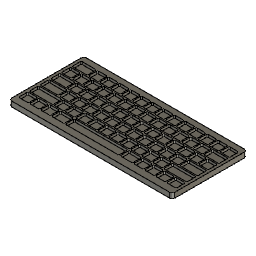
Week 3 HW Keyboard (Autodesk Fusion 360 design; units mm, degrees)
Autodesk Fusion 360 part; units mm, degrees
(part 1 of 2)
sketch "Key outlines" plane through (0, 0, 0) normal (0, 0, 1) x (1, 0, 0)
  spline S0 degree 3 poles (7.7819, -17.5295) (7.6676, -17.5295) (7.5745, -17.4364) (7.5745, -17.3224) knots 0 0 0 0 1 1 1 1
  line L0 (7.5745, -17.3224) -> (7.5745, -15.9198)
  spline S1 degree 3 poles (7.5745, -15.9198) (7.5745, -15.8059) (7.6676, -15.7127) (7.7819, -15.7127) knots 0 0 0 0 1 1 1 1
  line L1 (7.7819, -15.7127) -> (9.2724, -15.7127)
  spline S2 degree 3 poles (9.2724, -15.7127) (9.3864, -15.7127) (9.4795, -15.8059) (9.4795, -15.9198) knots 0 0 0 0 1 1 1 1
  line L2 (9.4795, -15.9198) -> (9.4795, -17.3224)
  spline S3 degree 3 poles (9.4795, -17.3224) (9.4795, -17.4364) (9.3864, -17.5295) (9.2724, -17.5295) knots 0 0 0 0 1 1 1 1
  line L3 (9.2724, -17.5295) -> (7.7819, -17.5295)
  spline S4 degree 3 poles (9.9243, -17.5295) (9.81, -17.5295) (9.7169, -17.4364) (9.7169, -17.3224) knots 0 0 0 0 1 1 1 1
  line L4 (9.7169, -17.3224) -> (9.7169, -15.9198)
  spline S5 degree 3 poles (9.7169, -15.9198) (9.7169, -15.8059) (9.81, -15.7127) (9.9243, -15.7127) knots 0 0 0 0 1 1 1 1
  line L5 (9.9243, -15.7127) -> (11.4148, -15.7127)
  spline S6 degree 3 poles (11.4148, -15.7127) (11.5291, -15.7127) (11.6219, -15.8059) (11.6219, -15.9198) knots 0 0 0 0 1 1 1 1
  line L6 (11.6219, -15.9198) -> (11.6219, -17.3224)
  spline S7 degree 3 poles (11.6219, -17.3224) (11.6219, -17.4364) (11.5291, -17.5295) (11.4148, -17.5295) knots 0 0 0 0 1 1 1 1
  line L7 (11.4148, -17.5295) -> (9.9243, -17.5295)
  spline S8 degree 3 poles (12.0668, -17.5295) (11.9525, -17.5295) (11.8593, -17.4364) (11.8593, -17.3224) knots 0 0 0 0 1 1 1 1
  line L8 (11.8593, -17.3224) -> (11.8593, -15.9198)
  spline S9 degree 3 poles (11.8593, -15.9198) (11.8593, -15.8059) (11.9525, -15.7127) (12.0668, -15.7127) knots 0 0 0 0 1 1 1 1
  line L9 (12.0668, -15.7127) -> (13.5572, -15.7127)
  spline S10 degree 3 poles (13.5572, -15.7127) (13.6716, -15.7127) (13.7643, -15.8059) (13.7643, -15.9198) knots 0 0 0 0 1 1 1 1
  line L10 (13.7643, -15.9198) -> (13.7643, -17.3224)
  spline S11 degree 3 poles (13.7643, -17.3224) (13.7643, -17.4364) (13.6716, -17.5295) (13.5572, -17.5295) knots 0 0 0 0 1 1 1 1
  line L11 (13.5572, -17.5295) -> (12.0668, -17.5295)
  spline S12 degree 3 poles (14.2092, -17.5295) (14.0949, -17.5295) (14.0017, -17.4364) (14.0017, -17.3224) knots 0 0 0 0 1 1 1 1
  line L12 (14.0017, -17.3224) -> (14.0017, -15.9198)
  spline S13 degree 3 poles (14.0017, -15.9198) (14.0017, -15.8059) (14.0949, -15.7127) (14.2092, -15.7127) knots 0 0 0 0 1 1 1 1
  line L13 (14.2092, -15.7127) -> (15.6997, -15.7127)
  spline S14 degree 3 poles (15.6997, -15.7127) (15.814, -15.7127) (15.9067, -15.8059) (15.9067, -15.9198) knots 0 0 0 0 1 1 1 1
  line L14 (15.9067, -15.9198) -> (15.9067, -17.3224)
  spline S15 degree 3 poles (15.9067, -17.3224) (15.9067, -17.4364) (15.814, -17.5295) (15.6997, -17.5295) knots 0 0 0 0 1 1 1 1
  line L15 (15.6997, -17.5295) -> (14.2092, -17.5295)
  spline S16 degree 3 poles (16.3516, -17.5295) (16.2373, -17.5295) (16.1445, -17.4364) (16.1445, -17.3224) knots 0 0 0 0 1 1 1 1
  line L16 (16.1445, -17.3224) -> (16.1445, -15.9198)
  spline S17 degree 3 poles (16.1445, -15.9198) (16.1445, -15.8059) (16.2373, -15.7127) (16.3516, -15.7127) knots 0 0 0 0 1 1 1 1
  line L17 (16.3516, -15.7127) -> (17.8421, -15.7127)
  spline S18 degree 3 poles (17.8421, -15.7127) (17.9564, -15.7127) (18.0492, -15.8059) (18.0492, -15.9198) knots 0 0 0 0 1 1 1 1
  line L18 (18.0492, -15.9198) -> (18.0492, -17.3224)
  spline S19 degree 3 poles (18.0492, -17.3224) (18.0492, -17.4364) (17.9564, -17.5295) (17.8421, -17.5295) knots 0 0 0 0 1 1 1 1
  line L19 (17.8421, -17.5295) -> (16.3516, -17.5295)
  spline S20 degree 3 poles (18.494, -17.5295) (18.3797, -17.5295) (18.2869, -17.4364) (18.2869, -17.3224) knots 0 0 0 0 1 1 1 1
  line L20 (18.2869, -17.3224) -> (18.2869, -15.9198)
  spline S21 degree 3 poles (18.2869, -15.9198) (18.2869, -15.8059) (18.3797, -15.7127) (18.494, -15.7127) knots 0 0 0 0 1 1 1 1
  line L21 (18.494, -15.7127) -> (19.9845, -15.7127)
  spline S22 degree 3 poles (19.9845, -15.7127) (20.0988, -15.7127) (20.1916, -15.8059) (20.1916, -15.9198) knots 0 0 0 0 1 1 1 1
  line L22 (20.1916, -15.9198) -> (20.1916, -17.3224)
  spline S23 degree 3 poles (20.1916, -17.3224) (20.1916, -17.4364) (20.0988, -17.5295) (19.9845, -17.5295) knots 0 0 0 0 1 1 1 1
  line L23 (19.9845, -17.5295) -> (18.494, -17.5295)
  spline S24 degree 3 poles (20.6364, -17.5295) (20.5221, -17.5295) (20.429, -17.4364) (20.429, -17.3224) knots 0 0 0 0 1 1 1 1
  line L24 (20.429, -17.3224) -> (20.429, -15.9198)
  spline S25 degree 3 poles (20.429, -15.9198) (20.429, -15.8059) (20.5221, -15.7127) (20.6364, -15.7127) knots 0 0 0 0 1 1 1 1
  line L25 (20.6364, -15.7127) -> (22.1269, -15.7127)
  spline S26 degree 3 poles (22.1269, -15.7127) (22.2412, -15.7127) (22.3344, -15.8059) (22.3344, -15.9198) knots 0 0 0 0 1 1 1 1
  line L26 (22.3344, -15.9198) -> (22.3344, -17.3224)
  spline S27 degree 3 poles (22.3344, -17.3224) (22.3344, -17.4364) (22.2412, -17.5295) (22.1269, -17.5295) knots 0 0 0 0 1 1 1 1
  line L27 (22.1269, -17.5295) -> (20.6364, -17.5295)
  spline S28 degree 3 poles (22.7789, -17.5295) (22.6646, -17.5295) (22.5714, -17.4364) (22.5714, -17.3224) knots 0 0 0 0 1 1 1 1
  line L28 (22.5714, -17.3224) -> (22.5714, -15.9198)
  spline S29 degree 3 poles (22.5714, -15.9198) (22.5714, -15.8059) (22.6646, -15.7127) (22.7789, -15.7127) knots 0 0 0 0 1 1 1 1
  line L29 (22.7789, -15.7127) -> (24.2693, -15.7127)
  spline S30 degree 3 poles (24.2693, -15.7127) (24.3836, -15.7127) (24.4768, -15.8059) (24.4768, -15.9198) knots 0 0 0 0 1 1 1 1
  line L30 (24.4768, -15.9198) -> (24.4768, -17.3224)
  spline S31 degree 3 poles (24.4768, -17.3224) (24.4768, -17.4364) (24.3836, -17.5295) (24.2693, -17.5295) knots 0 0 0 0 1 1 1 1
  line L31 (24.2693, -17.5295) -> (22.7789, -17.5295)
  spline S32 degree 3 poles (24.9216, -17.5295) (24.807, -17.5295) (24.7142, -17.4364) (24.7142, -17.3224) knots 0 0 0 0 1 1 1 1
  line L32 (24.7142, -17.3224) -> (24.7142, -15.9198)
  spline S33 degree 3 poles (24.7142, -15.9198) (24.7142, -15.8059) (24.807, -15.7127) (24.9216, -15.7127) knots 0 0 0 0 1 1 1 1
  line L33 (24.9216, -15.7127) -> (26.4118, -15.7127)
  spline S34 degree 3 poles (26.4118, -15.7127) (26.5261, -15.7127) (26.6192, -15.8059) (26.6192, -15.9198) knots 0 0 0 0 1 1 1 1
  line L34 (26.6192, -15.9198) -> (26.6192, -17.3224)
  spline S35 degree 3 poles (26.6192, -17.3224) (26.6192, -17.4364) (26.5261, -17.5295) (26.4118, -17.5295) knots 0 0 0 0 1 1 1 1
  line L35 (26.4118, -17.5295) -> (24.9216, -17.5295)
  spline S36 degree 3 poles (27.0641, -17.5295) (26.9498, -17.5295) (26.8566, -17.4364) (26.8566, -17.3224) knots 0 0 0 0 1 1 1 1
  line L36 (26.8566, -17.3224) -> (26.8566, -15.9198)
  spline S37 degree 3 poles (26.8566, -15.9198) (26.8566, -15.8059) (26.9498, -15.7127) (27.0641, -15.7127) knots 0 0 0 0 1 1 1 1
  line L37 (27.0641, -15.7127) -> (28.5542, -15.7127)
  spline S38 degree 3 poles (28.5542, -15.7127) (28.6688, -15.7127) (28.7616, -15.8059) (28.7616, -15.9198) knots 0 0 0 0 1 1 1 1
  line L38 (28.7616, -15.9198) -> (28.7616, -17.3224)
  spline S39 degree 3 poles (28.7616, -17.3224) (28.7616, -17.4364) (28.6688, -17.5295) (28.5542, -17.5295) knots 0 0 0 0 1 1 1 1
  line L39 (28.5542, -17.5295) -> (27.0641, -17.5295)
  spline S40 degree 3 poles (29.2061, -17.5295) (29.0922, -17.5295) (28.999, -17.4364) (28.999, -17.3224) knots 0 0 0 0 1 1 1 1
  line L40 (28.999, -17.3224) -> (28.999, -15.9198)
  spline S41 degree 3 poles (28.999, -15.9198) (28.999, -15.8059) (29.0922, -15.7127) (29.2061, -15.7127) knots 0 0 0 0 1 1 1 1
  line L41 (29.2061, -15.7127) -> (30.697, -15.7127)
  spline S42 degree 3 poles (30.697, -15.7127) (30.8109, -15.7127) (30.904, -15.8059) (30.904, -15.9198) knots 0 0 0 0 1 1 1 1
  line L42 (30.904, -15.9198) -> (30.904, -17.3224)
  spline S43 degree 3 poles (30.904, -17.3224) (30.904, -17.4364) (30.8109, -17.5295) (30.697, -17.5295) knots 0 0 0 0 1 1 1 1
  line L43 (30.697, -17.5295) -> (29.2061, -17.5295)
  spline S44 degree 3 poles (31.3485, -17.5295) (31.2342, -17.5295) (31.1415, -17.4364) (31.1415, -17.3224) knots 0 0 0 0 1 1 1 1
  line L44 (31.1415, -17.3224) -> (31.1415, -15.9198)
  spline S45 degree 3 poles (31.1415, -15.9198) (31.1415, -15.8059) (31.2342, -15.7127) (31.3485, -15.7127) knots 0 0 0 0 1 1 1 1
  line L45 (31.3485, -15.7127) -> (32.8394, -15.7127)
  spline S46 degree 3 poles (32.8394, -15.7127) (32.9533, -15.7127) (33.0465, -15.8059) (33.0465, -15.9198) knots 0 0 0 0 1 1 1 1
  line L46 (33.0465, -15.9198) -> (33.0465, -17.3224)
  spline S47 degree 3 poles (33.0465, -17.3224) (33.0465, -17.4364) (32.9533, -17.5295) (32.8394, -17.5295) knots 0 0 0 0 1 1 1 1
  line L47 (32.8394, -17.5295) -> (31.3485, -17.5295)
  spline S48 degree 3 poles (5.6392, -17.5295) (5.5252, -17.5295) (5.4321, -17.4364) (5.4321, -17.3224) knots 0 0 0 0 1 1 1 1
  line L48 (5.4321, -17.3224) -> (5.4321, -15.9198)
  spline S49 degree 3 poles (5.4321, -15.9198) (5.4321, -15.8059) (5.5252, -15.7127) (5.6392, -15.7127) knots 0 0 0 0 1 1 1 1
  line L49 (5.6392, -15.7127) -> (7.1296, -15.7127)
  spline S50 degree 3 poles (7.1296, -15.7127) (7.2443, -15.7127) (7.3371, -15.8059) (7.3371, -15.9198) knots 0 0 0 0 1 1 1 1
  line L50 (7.3371, -15.9198) -> (7.3371, -17.3224)
  spline S51 degree 3 poles (7.3371, -17.3224) (7.3371, -17.4364) (7.2443, -17.5295) (7.1296, -17.5295) knots 0 0 0 0 1 1 1 1
  line L51 (7.1296, -17.5295) -> (5.6392, -17.5295)
  spline S52 degree 3 poles (2.4208, -17.5295) (2.3068, -17.5295) (2.2137, -17.4364) (2.2137, -17.3224) knots 0 0 0 0 1 1 1 1
  line L52 (2.2137, -17.3224) -> (2.2137, -15.9198)
  spline S53 degree 3 poles (2.2137, -15.9198) (2.2137, -15.8059) (2.3068, -15.7127) (2.4208, -15.7127) knots 0 0 0 0 1 1 1 1
  line L53 (2.4208, -15.7127) -> (4.9876, -15.7127)
  spline S54 degree 3 poles (4.9876, -15.7127) (5.1015, -15.7127) (5.1947, -15.8059) (5.1947, -15.9198) knots 0 0 0 0 1 1 1 1
  line L54 (5.1947, -15.9198) -> (5.1947, -17.3224)
  spline S55 degree 3 poles (5.1947, -17.3224) (5.1947, -17.4364) (5.1015, -17.5295) (4.9876, -17.5295) knots 0 0 0 0 1 1 1 1
  line L55 (4.9876, -17.5295) -> (2.4208, -17.5295)
  spline S56 degree 3 poles (7.7819, -13.3526) (7.6676, -13.3526) (7.5745, -13.2595) (7.5745, -13.1456) knots 0 0 0 0 1 1 1 1
  line L56 (7.5745, -13.1456) -> (7.5745, -11.7433)
  spline S57 degree 3 poles (7.5745, -11.7433) (7.5745, -11.6286) (7.6676, -11.5358) (7.7819, -11.5358) knots 0 0 0 0 1 1 1 1
  line L57 (7.7819, -11.5358) -> (9.2724, -11.5358)
  spline S58 degree 3 poles (9.2724, -11.5358) (9.3864, -11.5358) (9.4795, -11.6286) (9.4795, -11.7433) knots 0 0 0 0 1 1 1 1
  line L58 (9.4795, -11.7433) -> (9.4795, -13.1456)
  spline S59 degree 3 poles (9.4795, -13.1456) (9.4795, -13.2595) (9.3864, -13.3526) (9.2724, -13.3526) knots 0 0 0 0 1 1 1 1
  line L59 (9.2724, -13.3526) -> (7.7819, -13.3526)
  spline S60 degree 3 poles (9.9243, -13.3526) (9.81, -13.3526) (9.7169, -13.2595) (9.7169, -13.1456) knots 0 0 0 0 1 1 1 1
  line L60 (9.7169, -13.1456) -> (9.7169, -11.7433)
  spline S61 degree 3 poles (9.7169, -11.7433) (9.7169, -11.6286) (9.81, -11.5358) (9.9243, -11.5358) knots 0 0 0 0 1 1 1 1
  line L61 (9.9243, -11.5358) -> (11.4148, -11.5358)
  spline S62 degree 3 poles (11.4148, -11.5358) (11.5291, -11.5358) (11.6219, -11.6286) (11.6219, -11.7433) knots 0 0 0 0 1 1 1 1
  line L62 (11.6219, -11.7433) -> (11.6219, -13.1456)
  spline S63 degree 3 poles (11.6219, -13.1456) (11.6219, -13.2595) (11.5291, -13.3526) (11.4148, -13.3526) knots 0 0 0 0 1 1 1 1
  line L63 (11.4148, -13.3526) -> (9.9243, -13.3526)
  spline S64 degree 3 poles (12.0668, -13.3526) (11.9525, -13.3526) (11.8593, -13.2595) (11.8593, -13.1456) knots 0 0 0 0 1 1 1 1
  line L64 (11.8593, -13.1456) -> (11.8593, -11.7433)
  spline S65 degree 3 poles (11.8593, -11.7433) (11.8593, -11.6286) (11.9525, -11.5358) (12.0668, -11.5358) knots 0 0 0 0 1 1 1 1
  line L65 (12.0668, -11.5358) -> (13.5572, -11.5358)
  spline S66 degree 3 poles (13.5572, -11.5358) (13.6716, -11.5358) (13.7643, -11.6286) (13.7643, -11.7433) knots 0 0 0 0 1 1 1 1
  line L66 (13.7643, -11.7433) -> (13.7643, -13.1456)
  spline S67 degree 3 poles (13.7643, -13.1456) (13.7643, -13.2595) (13.6716, -13.3526) (13.5572, -13.3526) knots 0 0 0 0 1 1 1 1
  line L67 (13.5572, -13.3526) -> (12.0668, -13.3526)
  spline S68 degree 3 poles (14.2092, -13.3526) (14.0949, -13.3526) (14.0017, -13.2595) (14.0017, -13.1456) knots 0 0 0 0 1 1 1 1
  line L68 (14.0017, -13.1456) -> (14.0017, -11.7433)
  spline S69 degree 3 poles (14.0017, -11.7433) (14.0017, -11.6286) (14.0949, -11.5358) (14.2092, -11.5358) knots 0 0 0 0 1 1 1 1
  line L69 (14.2092, -11.5358) -> (15.6997, -11.5358)
  spline S70 degree 3 poles (15.6997, -11.5358) (15.814, -11.5358) (15.9067, -11.6286) (15.9067, -11.7433) knots 0 0 0 0 1 1 1 1
  line L70 (15.9067, -11.7433) -> (15.9067, -13.1456)
  spline S71 degree 3 poles (15.9067, -13.1456) (15.9067, -13.2595) (15.814, -13.3526) (15.6997, -13.3526) knots 0 0 0 0 1 1 1 1
  line L71 (15.6997, -13.3526) -> (14.2092, -13.3526)
  spline S72 degree 3 poles (16.3516, -13.3526) (16.2373, -13.3526) (16.1445, -13.2595) (16.1445, -13.1456) knots 0 0 0 0 1 1 1 1
  line L72 (16.1445, -13.1456) -> (16.1445, -11.7433)
  spline S73 degree 3 poles (16.1445, -11.7433) (16.1445, -11.6286) (16.2373, -11.5358) (16.3516, -11.5358) knots 0 0 0 0 1 1 1 1
  line L73 (16.3516, -11.5358) -> (17.8421, -11.5358)
  spline S74 degree 3 poles (17.8421, -11.5358) (17.9564, -11.5358) (18.0492, -11.6286) (18.0492, -11.7433) knots 0 0 0 0 1 1 1 1
  line L74 (18.0492, -11.7433) -> (18.0492, -13.1456)
  spline S75 degree 3 poles (18.0492, -13.1456) (18.0492, -13.2595) (17.9564, -13.3526) (17.8421, -13.3526) knots 0 0 0 0 1 1 1 1
  line L75 (17.8421, -13.3526) -> (16.3516, -13.3526)
  spline S76 degree 3 poles (18.494, -13.3526) (18.3797, -13.3526) (18.2869, -13.2595) (18.2869, -13.1456) knots 0 0 0 0 1 1 1 1
  line L76 (18.2869, -13.1456) -> (18.2869, -11.7433)
  spline S77 degree 3 poles (18.2869, -11.7433) (18.2869, -11.6286) (18.3797, -11.5358) (18.494, -11.5358) knots 0 0 0 0 1 1 1 1
  line L77 (18.494, -11.5358) -> (19.9845, -11.5358)
  spline S78 degree 3 poles (19.9845, -11.5358) (20.0988, -11.5358) (20.1916, -11.6286) (20.1916, -11.7433) knots 0 0 0 0 1 1 1 1
  line L78 (20.1916, -11.7433) -> (20.1916, -13.1456)
  spline S79 degree 3 poles (20.1916, -13.1456) (20.1916, -13.2595) (20.0988, -13.3526) (19.9845, -13.3526) knots 0 0 0 0 1 1 1 1
  line L79 (19.9845, -13.3526) -> (18.494, -13.3526)
  spline S80 degree 3 poles (20.6364, -13.3526) (20.5221, -13.3526) (20.429, -13.2595) (20.429, -13.1456) knots 0 0 0 0 1 1 1 1
  line L80 (20.429, -13.1456) -> (20.429, -11.7433)
  spline S81 degree 3 poles (20.429, -11.7433) (20.429, -11.6286) (20.5221, -11.5358) (20.6364, -11.5358) knots 0 0 0 0 1 1 1 1
  line L81 (20.6364, -11.5358) -> (22.1269, -11.5358)
  spline S82 degree 3 poles (22.1269, -11.5358) (22.2412, -11.5358) (22.3344, -11.6286) (22.3344, -11.7433) knots 0 0 0 0 1 1 1 1
  line L82 (22.3344, -11.7433) -> (22.3344, -13.1456)
  spline S83 degree 3 poles (22.3344, -13.1456) (22.3344, -13.2595) (22.2412, -13.3526) (22.1269, -13.3526) knots 0 0 0 0 1 1 1 1
  line L83 (22.1269, -13.3526) -> (20.6364, -13.3526)
  spline S84 degree 3 poles (22.7789, -13.3526) (22.6646, -13.3526) (22.5714, -13.2595) (22.5714, -13.1456) knots 0 0 0 0 1 1 1 1
  line L84 (22.5714, -13.1456) -> (22.5714, -11.7433)
  spline S85 degree 3 poles (22.5714, -11.7433) (22.5714, -11.6286) (22.6646, -11.5358) (22.7789, -11.5358) knots 0 0 0 0 1 1 1 1
  line L85 (22.7789, -11.5358) -> (24.2693, -11.5358)
  spline S86 degree 3 poles (24.2693, -11.5358) (24.3836, -11.5358) (24.4768, -11.6286) (24.4768, -11.7433) knots 0 0 0 0 1 1 1 1
  line L86 (24.4768, -11.7433) -> (24.4768, -13.1456)
  spline S87 degree 3 poles (24.4768, -13.1456) (24.4768, -13.2595) (24.3836, -13.3526) (24.2693, -13.3526) knots 0 0 0 0 1 1 1 1
  line L87 (24.2693, -13.3526) -> (22.7789, -13.3526)
  spline S88 degree 3 poles (24.9216, -13.3526) (24.807, -13.3526) (24.7142, -13.2595) (24.7142, -13.1456) knots 0 0 0 0 1 1 1 1
  line L88 (24.7142, -13.1456) -> (24.7142, -11.7433)
  spline S89 degree 3 poles (24.7142, -11.7433) (24.7142, -11.6286) (24.807, -11.5358) (24.9216, -11.5358) knots 0 0 0 0 1 1 1 1
  line L89 (24.9216, -11.5358) -> (26.4118, -11.5358)
  spline S90 degree 3 poles (26.4118, -11.5358) (26.5261, -11.5358) (26.6192, -11.6286) (26.6192, -11.7433) knots 0 0 0 0 1 1 1 1
  line L90 (26.6192, -11.7433) -> (26.6192, -13.1456)
  spline S91 degree 3 poles (26.6192, -13.1456) (26.6192, -13.2595) (26.5261, -13.3526) (26.4118, -13.3526) knots 0 0 0 0 1 1 1 1
  line L91 (26.4118, -13.3526) -> (24.9216, -13.3526)
  spline S92 degree 3 poles (27.0641, -13.3526) (26.9498, -13.3526) (26.8566, -13.2595) (26.8566, -13.1456) knots 0 0 0 0 1 1 1 1
  line L92 (26.8566, -13.1456) -> (26.8566, -11.7433)
  spline S93 degree 3 poles (26.8566, -11.7433) (26.8566, -11.6286) (26.9498, -11.5358) (27.0641, -11.5358) knots 0 0 0 0 1 1 1 1
  line L93 (27.0641, -11.5358) -> (28.5542, -11.5358)
  spline S94 degree 3 poles (28.5542, -11.5358) (28.6688, -11.5358) (28.7616, -11.6286) (28.7616, -11.7433) knots 0 0 0 0 1 1 1 1
  line L94 (28.7616, -11.7433) -> (28.7616, -13.1456)
  spline S95 degree 3 poles (28.7616, -13.1456) (28.7616, -13.2595) (28.6688, -13.3526) (28.5542, -13.3526) knots 0 0 0 0 1 1 1 1
  line L95 (28.5542, -13.3526) -> (27.0641, -13.3526)
  spline S96 degree 3 poles (29.2061, -13.3526) (29.0922, -13.3526) (28.999, -13.2595) (28.999, -13.1456) knots 0 0 0 0 1 1 1 1
  line L96 (28.999, -13.1456) -> (28.999, -11.7433)
  spline S97 degree 3 poles (28.999, -11.7433) (28.999, -11.6286) (29.0922, -11.5358) (29.2061, -11.5358) knots 0 0 0 0 1 1 1 1
  line L97 (29.2061, -11.5358) -> (30.697, -11.5358)
  spline S98 degree 3 poles (30.697, -11.5358) (30.8109, -11.5358) (30.904, -11.6286) (30.904, -11.7433) knots 0 0 0 0 1 1 1 1
  line L98 (30.904, -11.7433) -> (30.904, -13.1456)
  spline S99 degree 3 poles (30.904, -13.1456) (30.904, -13.2595) (30.8109, -13.3526) (30.697, -13.3526) knots 0 0 0 0 1 1 1 1
  line L99 (30.697, -13.3526) -> (29.2061, -13.3526)
  spline S100 degree 3 poles (31.3485, -13.3526) (31.2342, -13.3526) (31.1415, -13.2595) (31.1415, -13.1456) knots 0 0 0 0 1 1 1 1
  line L100 (31.1415, -13.1456) -> (31.1415, -11.7433)
  spline S101 degree 3 poles (31.1415, -11.7433) (31.1415, -11.6286) (31.2342, -11.5358) (31.3485, -11.5358) knots 0 0 0 0 1 1 1 1
  line L101 (31.3485, -11.5358) -> (32.8394, -11.5358)
  spline S102 degree 3 poles (32.8394, -11.5358) (32.9533, -11.5358) (33.0465, -11.6286) (33.0465, -11.7433) knots 0 0 0 0 1 1 1 1
  line L102 (33.0465, -11.7433) -> (33.0465, -13.1456)
  spline S103 degree 3 poles (33.0465, -13.1456) (33.0465, -13.2595) (32.9533, -13.3526) (32.8394, -13.3526) knots 0 0 0 0 1 1 1 1
  line L103 (32.8394, -13.3526) -> (31.3485, -13.3526)
  spline S104 degree 3 poles (5.6392, -13.3526) (5.5252, -13.3526) (5.4321, -13.2595) (5.4321, -13.1456) knots 0 0 0 0 1 1 1 1
  line L104 (5.4321, -13.1456) -> (5.4321, -11.7433)
  spline S105 degree 3 poles (5.4321, -11.7433) (5.4321, -11.6286) (5.5252, -11.5358) (5.6392, -11.5358) knots 0 0 0 0 1 1 1 1
  line L105 (5.6392, -11.5358) -> (7.1296, -11.5358)
  spline S106 degree 3 poles (7.1296, -11.5358) (7.2443, -11.5358) (7.3371, -11.6286) (7.3371, -11.7433) knots 0 0 0 0 1 1 1 1
  line L106 (7.3371, -11.7433) -> (7.3371, -13.1456)
  spline S107 degree 3 poles (7.3371, -13.1456) (7.3371, -13.2595) (7.2443, -13.3526) (7.1296, -13.3526) knots 0 0 0 0 1 1 1 1
  line L107 (7.1296, -13.3526) -> (5.6392, -13.3526)
  spline S108 degree 3 poles (2.4208, -13.3526) (2.3068, -13.3526) (2.2137, -13.2595) (2.2137, -13.1456) knots 0 0 0 0 1 1 1 1
  line L108 (2.2137, -13.1456) -> (2.2137, -11.7433)
  spline S109 degree 3 poles (2.2137, -11.7433) (2.2137, -11.6286) (2.3068, -11.5358) (2.4208, -11.5358) knots 0 0 0 0 1 1 1 1
  line L109 (2.4208, -11.5358) -> (4.9876, -11.5358)
  spline S110 degree 3 poles (4.9876, -11.5358) (5.1015, -11.5358) (5.1947, -11.6286) (5.1947, -11.7433) knots 0 0 0 0 1 1 1 1
  line L110 (5.1947, -11.7433) -> (5.1947, -13.1456)
  spline S111 degree 3 poles (5.1947, -13.1456) (5.1947, -13.2595) (5.1015, -13.3526) (4.9876, -13.3526) knots 0 0 0 0 1 1 1 1
  line L111 (4.9876, -13.3526) -> (2.4208, -13.3526)
  spline S112 degree 3 poles (6.706, -15.4411) (6.5917, -15.4411) (6.4985, -15.3479) (6.4985, -15.234) knots 0 0 0 0 1 1 1 1
  line L112 (6.4985, -15.234) -> (6.4985, -13.8317)
  spline S113 degree 3 poles (6.4985, -13.8317) (6.4985, -13.7174) (6.5917, -13.6243) (6.706, -13.6243) knots 0 0 0 0 1 1 1 1
  line L113 (6.706, -13.6243) -> (8.1964, -13.6243)
  spline S114 degree 3 poles (8.1964, -13.6243) (8.3107, -13.6243) (8.4035, -13.7174) (8.4035, -13.8317) knots 0 0 0 0 1 1 1 1
  line L114 (8.4035, -13.8317) -> (8.4035, -15.234)
  spline S115 degree 3 poles (8.4035, -15.234) (8.4035, -15.3479) (8.3107, -15.4411) (8.1964, -15.4411) knots 0 0 0 0 1 1 1 1
  line L115 (8.1964, -15.4411) -> (6.706, -15.4411)
  spline S116 degree 3 poles (8.8484, -15.4411) (8.7341, -15.4411) (8.6409, -15.3479) (8.6409, -15.234) knots 0 0 0 0 1 1 1 1
  line L116 (8.6409, -15.234) -> (8.6409, -13.8317)
  spline S117 degree 3 poles (8.6409, -13.8317) (8.6409, -13.7174) (8.7341, -13.6243) (8.8484, -13.6243) knots 0 0 0 0 1 1 1 1
  line L117 (8.8484, -13.6243) -> (10.3389, -13.6243)
  spline S118 degree 3 poles (10.3389, -13.6243) (10.4532, -13.6243) (10.5459, -13.7174) (10.5459, -13.8317) knots 0 0 0 0 1 1 1 1
  line L118 (10.5459, -13.8317) -> (10.5459, -15.234)
  spline S119 degree 3 poles (10.5459, -15.234) (10.5459, -15.3479) (10.4532, -15.4411) (10.3389, -15.4411) knots 0 0 0 0 1 1 1 1
  line L119 (10.3389, -15.4411) -> (8.8484, -15.4411)
  spline S120 degree 3 poles (10.9908, -15.4411) (10.8765, -15.4411) (10.7834, -15.3479) (10.7834, -15.234) knots 0 0 0 0 1 1 1 1
  line L120 (10.7834, -15.234) -> (10.7834, -13.8317)
  spline S121 degree 3 poles (10.7834, -13.8317) (10.7834, -13.7174) (10.8765, -13.6243) (10.9908, -13.6243) knots 0 0 0 0 1 1 1 1
  line L121 (10.9908, -13.6243) -> (12.4813, -13.6243)
  spline S122 degree 3 poles (12.4813, -13.6243) (12.5956, -13.6243) (12.6884, -13.7174) (12.6884, -13.8317) knots 0 0 0 0 1 1 1 1
  line L122 (12.6884, -13.8317) -> (12.6884, -15.234)
  spline S123 degree 3 poles (12.6884, -15.234) (12.6884, -15.3479) (12.5956, -15.4411) (12.4813, -15.4411) knots 0 0 0 0 1 1 1 1
  line L123 (12.4813, -15.4411) -> (10.9908, -15.4411)
  spline S124 degree 3 poles (13.1332, -15.4411) (13.0189, -15.4411) (12.9261, -15.3479) (12.9261, -15.234) knots 0 0 0 0 1 1 1 1
  line L124 (12.9261, -15.234) -> (12.9261, -13.8317)
  spline S125 degree 3 poles (12.9261, -13.8317) (12.9261, -13.7174) (13.0189, -13.6243) (13.1332, -13.6243) knots 0 0 0 0 1 1 1 1
  line L125 (13.1332, -13.6243) -> (14.6237, -13.6243)
  spline S126 degree 3 poles (14.6237, -13.6243) (14.738, -13.6243) (14.8311, -13.7174) (14.8311, -13.8317) knots 0 0 0 0 1 1 1 1
  line L126 (14.8311, -13.8317) -> (14.8311, -15.234)
  spline S127 degree 3 poles (14.8311, -15.234) (14.8311, -15.3479) (14.738, -15.4411) (14.6237, -15.4411) knots 0 0 0 0 1 1 1 1
  line L127 (14.6237, -15.4411) -> (13.1332, -15.4411)
  spline S128 degree 3 poles (15.2756, -15.4411) (15.1613, -15.4411) (15.0682, -15.3479) (15.0682, -15.234) knots 0 0 0 0 1 1 1 1
  line L128 (15.0682, -15.234) -> (15.0682, -13.8317)
  spline S129 degree 3 poles (15.0682, -13.8317) (15.0682, -13.7174) (15.1613, -13.6243) (15.2756, -13.6243) knots 0 0 0 0 1 1 1 1
  line L129 (15.2756, -13.6243) -> (16.7661, -13.6243)
  spline S130 degree 3 poles (16.7661, -13.6243) (16.8804, -13.6243) (16.9732, -13.7174) (16.9732, -13.8317) knots 0 0 0 0 1 1 1 1
  line L130 (16.9732, -13.8317) -> (16.9732, -15.234)
  spline S131 degree 3 poles (16.9732, -15.234) (16.9732, -15.3479) (16.8804, -15.4411) (16.7661, -15.4411) knots 0 0 0 0 1 1 1 1
  line L131 (16.7661, -15.4411) -> (15.2756, -15.4411)
  spline S132 degree 3 poles (17.418, -15.4411) (17.3037, -15.4411) (17.211, -15.3479) (17.211, -15.234) knots 0 0 0 0 1 1 1 1
  line L132 (17.211, -15.234) -> (17.211, -13.8317)
  spline S133 degree 3 poles (17.211, -13.8317) (17.211, -13.7174) (17.3037, -13.6243) (17.418, -13.6243) knots 0 0 0 0 1 1 1 1
  line L133 (17.418, -13.6243) -> (18.9085, -13.6243)
  spline S134 degree 3 poles (18.9085, -13.6243) (19.0228, -13.6243) (19.116, -13.7174) (19.116, -13.8317) knots 0 0 0 0 1 1 1 1
  line L134 (19.116, -13.8317) -> (19.116, -15.234)
  spline S135 degree 3 poles (19.116, -15.234) (19.116, -15.3479) (19.0228, -15.4411) (18.9085, -15.4411) knots 0 0 0 0 1 1 1 1
  line L135 (18.9085, -15.4411) -> (17.418, -15.4411)
  spline S136 degree 3 poles (19.5605, -15.4411) (19.4462, -15.4411) (19.353, -15.3479) (19.353, -15.234) knots 0 0 0 0 1 1 1 1
  line L136 (19.353, -15.234) -> (19.353, -13.8317)
  spline S137 degree 3 poles (19.353, -13.8317) (19.353, -13.7174) (19.4462, -13.6243) (19.5605, -13.6243) knots 0 0 0 0 1 1 1 1
  line L137 (19.5605, -13.6243) -> (21.051, -13.6243)
  spline S138 degree 3 poles (21.051, -13.6243) (21.1653, -13.6243) (21.2584, -13.7174) (21.2584, -13.8317) knots 0 0 0 0 1 1 1 1
  line L138 (21.2584, -13.8317) -> (21.2584, -15.234)
  spline S139 degree 3 poles (21.2584, -15.234) (21.2584, -15.3479) (21.1653, -15.4411) (21.051, -15.4411) knots 0 0 0 0 1 1 1 1
  line L139 (21.051, -15.4411) -> (19.5605, -15.4411)
  spline S140 degree 3 poles (21.7032, -15.4411) (21.5886, -15.4411) (21.4958, -15.3479) (21.4958, -15.234) knots 0 0 0 0 1 1 1 1
  line L140 (21.4958, -15.234) -> (21.4958, -13.8317)
  spline S141 degree 3 poles (21.4958, -13.8317) (21.4958, -13.7174) (21.5886, -13.6243) (21.7032, -13.6243) knots 0 0 0 0 1 1 1 1
  line L141 (21.7032, -13.6243) -> (23.1934, -13.6243)
  spline S142 degree 3 poles (23.1934, -13.6243) (23.3077, -13.6243) (23.4008, -13.7174) (23.4008, -13.8317) knots 0 0 0 0 1 1 1 1
  line L142 (23.4008, -13.8317) -> (23.4008, -15.234)
  spline S143 degree 3 poles (23.4008, -15.234) (23.4008, -15.3479) (23.3077, -15.4411) (23.1934, -15.4411) knots 0 0 0 0 1 1 1 1
  line L143 (23.1934, -15.4411) -> (21.7032, -15.4411)
  spline S144 degree 3 poles (23.8457, -15.4411) (23.7314, -15.4411) (23.6382, -15.3479) (23.6382, -15.234) knots 0 0 0 0 1 1 1 1
  line L144 (23.6382, -15.234) -> (23.6382, -13.8317)
  spline S145 degree 3 poles (23.6382, -13.8317) (23.6382, -13.7174) (23.7314, -13.6243) (23.8457, -13.6243) knots 0 0 0 0 1 1 1 1
  line L145 (23.8457, -13.6243) -> (25.3358, -13.6243)
  spline S146 degree 3 poles (25.3358, -13.6243) (25.4504, -13.6243) (25.5432, -13.7174) (25.5432, -13.8317) knots 0 0 0 0 1 1 1 1
  line L146 (25.5432, -13.8317) -> (25.5432, -15.234)
  spline S147 degree 3 poles (25.5432, -15.234) (25.5432, -15.3479) (25.4504, -15.4411) (25.3358, -15.4411) knots 0 0 0 0 1 1 1 1
  line L147 (25.3358, -15.4411) -> (23.8457, -15.4411)
  spline S148 degree 3 poles (25.9877, -15.4411) (25.8738, -15.4411) (25.7806, -15.3479) (25.7806, -15.234) knots 0 0 0 0 1 1 1 1
  line L148 (25.7806, -15.234) -> (25.7806, -13.8317)
  spline S149 degree 3 poles (25.7806, -13.8317) (25.7806, -13.7174) (25.8738, -13.6243) (25.9877, -13.6243) knots 0 0 0 0 1 1 1 1
  line L149 (25.9877, -13.6243) -> (27.4786, -13.6243)
  spline S150 degree 3 poles (27.4786, -13.6243) (27.5925, -13.6243) (27.6856, -13.7174) (27.6856, -13.8317) knots 0 0 0 0 1 1 1 1
  line L150 (27.6856, -13.8317) -> (27.6856, -15.234)
  spline S151 degree 3 poles (27.6856, -15.234) (27.6856, -15.3479) (27.5925, -15.4411) (27.4786, -15.4411) knots 0 0 0 0 1 1 1 1
  line L151 (27.4786, -15.4411) -> (25.9877, -15.4411)
  spline S152 degree 3 poles (28.1301, -15.4411) (28.0158, -15.4411) (27.9231, -15.3479) (27.9231, -15.234) knots 0 0 0 0 1 1 1 1
  line L152 (27.9231, -15.234) -> (27.9231, -13.8317)
  spline S153 degree 3 poles (27.9231, -13.8317) (27.9231, -13.7174) (28.0158, -13.6243) (28.1301, -13.6243) knots 0 0 0 0 1 1 1 1
  line L153 (28.1301, -13.6243) -> (29.621, -13.6243)
  spline S154 degree 3 poles (29.621, -13.6243) (29.7349, -13.6243) (29.8281, -13.7174) (29.8281, -13.8317) knots 0 0 0 0 1 1 1 1
  line L154 (29.8281, -13.8317) -> (29.8281, -15.234)
  spline S155 degree 3 poles (29.8281, -15.234) (29.8281, -15.3479) (29.7349, -15.4411) (29.621, -15.4411) knots 0 0 0 0 1 1 1 1
  line L155 (29.621, -15.4411) -> (28.1301, -15.4411)
  spline S156 degree 3 poles (30.2729, -15.4411) (30.1583, -15.4411) (30.0655, -15.3479) (30.0655, -15.234) knots 0 0 0 0 1 1 1 1
  line L156 (30.0655, -15.234) -> (30.0655, -13.8317)
  spline S157 degree 3 poles (30.0655, -13.8317) (30.0655, -13.7174) (30.1583, -13.6243) (30.2729, -13.6243) knots 0 0 0 0 1 1 1 1
  line L157 (30.2729, -13.6243) -> (32.8394, -13.6243)
  spline S158 degree 3 poles (32.8394, -13.6243) (32.9533, -13.6243) (33.0465, -13.7174) (33.0465, -13.8317) knots 0 0 0 0 1 1 1 1
  line L158 (33.0465, -13.8317) -> (33.0465, -15.234)
  spline S159 degree 3 poles (33.0465, -15.234) (33.0465, -15.3479) (32.9533, -15.4411) (32.8394, -15.4411) knots 0 0 0 0 1 1 1 1
  line L159 (32.8394, -15.4411) -> (30.2729, -15.4411)
  spline S160 degree 3 poles (4.5635, -15.4411) (4.4492, -15.4411) (4.3561, -15.3479) (4.3561, -15.234) knots 0 0 0 0 1 1 1 1
  line L160 (4.3561, -15.234) -> (4.3561, -13.8317)
  spline S161 degree 3 poles (4.3561, -13.8317) (4.3561, -13.7174) (4.4492, -13.6243) (4.5635, -13.6243) knots 0 0 0 0 1 1 1 1
  line L161 (4.5635, -13.6243) -> (6.054, -13.6243)
  spline S162 degree 3 poles (6.054, -13.6243) (6.168, -13.6243) (6.2611, -13.7174) (6.2611, -13.8317) knots 0 0 0 0 1 1 1 1
  line L162 (6.2611, -13.8317) -> (6.2611, -15.234)
  spline S163 degree 3 poles (6.2611, -15.234) (6.2611, -15.3479) (6.168, -15.4411) (6.054, -15.4411) knots 0 0 0 0 1 1 1 1
  line L163 (6.054, -15.4411) -> (4.5635, -15.4411)
  spline S164 degree 3 poles (2.4208, -15.4411) (2.3068, -15.4411) (2.2137, -15.3479) (2.2137, -15.234) knots 0 0 0 0 1 1 1 1
  line L164 (2.2137, -15.234) -> (2.2137, -13.8317)
  spline S165 degree 3 poles (2.2137, -13.8317) (2.2137, -13.7174) (2.3068, -13.6243) (2.4208, -13.6243) knots 0 0 0 0 1 1 1 1
  line L165 (2.4208, -13.6243) -> (3.9112, -13.6243)
  spline S166 degree 3 poles (3.9112, -13.6243) (4.0259, -13.6243) (4.1187, -13.7174) (4.1187, -13.8317) knots 0 0 0 0 1 1 1 1
  line L166 (4.1187, -13.8317) -> (4.1187, -15.234)
  spline S167 degree 3 poles (4.1187, -15.234) (4.1187, -15.3479) (4.0259, -15.4411) (3.9112, -15.4411) knots 0 0 0 0 1 1 1 1
  line L167 (3.9112, -15.4411) -> (2.4208, -15.4411)
  spline S168 degree 3 poles (8.3111, -19.618) (8.1968, -19.618) (8.1037, -19.5252) (8.1037, -19.4105) knots 0 0 0 0 1 1 1 1
  line L168 (8.1037, -19.4105) -> (8.1037, -18.0086)
  spline S169 degree 3 poles (8.1037, -18.0086) (8.1037, -17.8943) (8.1968, -17.8012) (8.3111, -17.8012) knots 0 0 0 0 1 1 1 1
  line L169 (8.3111, -17.8012) -> (9.8016, -17.8012)
  spline S170 degree 3 poles (9.8016, -17.8012) (9.9155, -17.8012) (10.0087, -17.8943) (10.0087, -18.0086) knots 0 0 0 0 1 1 1 1
  line L170 (10.0087, -18.0086) -> (10.0087, -19.4105)
  spline S171 degree 3 poles (10.0087, -19.4105) (10.0087, -19.5252) (9.9155, -19.618) (9.8016, -19.618) knots 0 0 0 0 1 1 1 1
  line L171 (9.8016, -19.618) -> (8.3111, -19.618)
  spline S172 degree 3 poles (10.4535, -19.618) (10.3392, -19.618) (10.2461, -19.5252) (10.2461, -19.4105) knots 0 0 0 0 1 1 1 1
  line L172 (10.2461, -19.4105) -> (10.2461, -18.0086)
  spline S173 degree 3 poles (10.2461, -18.0086) (10.2461, -17.8943) (10.3392, -17.8012) (10.4535, -17.8012) knots 0 0 0 0 1 1 1 1
  line L173 (10.4535, -17.8012) -> (11.944, -17.8012)
  spline S174 degree 3 poles (11.944, -17.8012) (12.0583, -17.8012) (12.1511, -17.8943) (12.1511, -18.0086) knots 0 0 0 0 1 1 1 1
  line L174 (12.1511, -18.0086) -> (12.1511, -19.4105)
  spline S175 degree 3 poles (12.1511, -19.4105) (12.1511, -19.5252) (12.0583, -19.618) (11.944, -19.618) knots 0 0 0 0 1 1 1 1
  line L175 (11.944, -19.618) -> (10.4535, -19.618)
  spline S176 degree 3 poles (12.5959, -19.618) (12.4816, -19.618) (12.3885, -19.5252) (12.3885, -19.4105) knots 0 0 0 0 1 1 1 1
  line L176 (12.3885, -19.4105) -> (12.3885, -18.0086)
  spline S177 degree 3 poles (12.3885, -18.0086) (12.3885, -17.8943) (12.4816, -17.8012) (12.5959, -17.8012) knots 0 0 0 0 1 1 1 1
  line L177 (12.5959, -17.8012) -> (14.0864, -17.8012)
  spline S178 degree 3 poles (14.0864, -17.8012) (14.2007, -17.8012) (14.2935, -17.8943) (14.2935, -18.0086) knots 0 0 0 0 1 1 1 1
  line L178 (14.2935, -18.0086) -> (14.2935, -19.4105)
  spline S179 degree 3 poles (14.2935, -19.4105) (14.2935, -19.5252) (14.2007, -19.618) (14.0864, -19.618) knots 0 0 0 0 1 1 1 1
  line L179 (14.0864, -19.618) -> (12.5959, -19.618)
  spline S180 degree 3 poles (14.7383, -19.618) (14.624, -19.618) (14.5309, -19.5252) (14.5309, -19.4105) knots 0 0 0 0 1 1 1 1
  line L180 (14.5309, -19.4105) -> (14.5309, -18.0086)
  spline S181 degree 3 poles (14.5309, -18.0086) (14.5309, -17.8943) (14.624, -17.8012) (14.7383, -17.8012) knots 0 0 0 0 1 1 1 1
  line L181 (14.7383, -17.8012) -> (16.2288, -17.8012)
  spline S182 degree 3 poles (16.2288, -17.8012) (16.3431, -17.8012) (16.4359, -17.8943) (16.4359, -18.0086) knots 0 0 0 0 1 1 1 1
  line L182 (16.4359, -18.0086) -> (16.4359, -19.4105)
  spline S183 degree 3 poles (16.4359, -19.4105) (16.4359, -19.5252) (16.3431, -19.618) (16.2288, -19.618) knots 0 0 0 0 1 1 1 1
  line L183 (16.2288, -19.618) -> (14.7383, -19.618)
  spline S184 degree 3 poles (16.8808, -19.618) (16.7665, -19.618) (16.6737, -19.5252) (16.6737, -19.4105) knots 0 0 0 0 1 1 1 1
  line L184 (16.6737, -19.4105) -> (16.6737, -18.0086)
  spline S185 degree 3 poles (16.6737, -18.0086) (16.6737, -17.8943) (16.7665, -17.8012) (16.8808, -17.8012) knots 0 0 0 0 1 1 1 1
  line L185 (16.8808, -17.8012) -> (18.3713, -17.8012)
  spline S186 degree 3 poles (18.3713, -17.8012) (18.4856, -17.8012) (18.5783, -17.8943) (18.5783, -18.0086) knots 0 0 0 0 1 1 1 1
  line L186 (18.5783, -18.0086) -> (18.5783, -19.4105)
  spline S187 degree 3 poles (18.5783, -19.4105) (18.5783, -19.5252) (18.4856, -19.618) (18.3713, -19.618) knots 0 0 0 0 1 1 1 1
  line L187 (18.3713, -19.618) -> (16.8808, -19.618)
  spline S188 degree 3 poles (19.0232, -19.618) (18.9089, -19.618) (18.8161, -19.5252) (18.8161, -19.4105) knots 0 0 0 0 1 1 1 1
  line L188 (18.8161, -19.4105) -> (18.8161, -18.0086)
  spline S189 degree 3 poles (18.8161, -18.0086) (18.8161, -17.8943) (18.9089, -17.8012) (19.0232, -17.8012) knots 0 0 0 0 1 1 1 1
  line L189 (19.0232, -17.8012) -> (20.5137, -17.8012)
  spline S190 degree 3 poles (20.5137, -17.8012) (20.628, -17.8012) (20.7208, -17.8943) (20.7208, -18.0086) knots 0 0 0 0 1 1 1 1
  line L190 (20.7208, -18.0086) -> (20.7208, -19.4105)
  spline S191 degree 3 poles (20.7208, -19.4105) (20.7208, -19.5252) (20.628, -19.618) (20.5137, -19.618) knots 0 0 0 0 1 1 1 1
  line L191 (20.5137, -19.618) -> (19.0232, -19.618)
  spline S192 degree 3 poles (21.1656, -19.618) (21.0513, -19.618) (20.9582, -19.5252) (20.9582, -19.4105) knots 0 0 0 0 1 1 1 1
  line L192 (20.9582, -19.4105) -> (20.9582, -18.0086)
  spline S193 degree 3 poles (20.9582, -18.0086) (20.9582, -17.8943) (21.0513, -17.8012) (21.1656, -17.8012) knots 0 0 0 0 1 1 1 1
  line L193 (21.1656, -17.8012) -> (22.6561, -17.8012)
  spline S194 degree 3 poles (22.6561, -17.8012) (22.7704, -17.8012) (22.8635, -17.8943) (22.8635, -18.0086) knots 0 0 0 0 1 1 1 1
  line L194 (22.8635, -18.0086) -> (22.8635, -19.4105)
  spline S195 degree 3 poles (22.8635, -19.4105) (22.8635, -19.5252) (22.7704, -19.618) (22.6561, -19.618) knots 0 0 0 0 1 1 1 1
  line L195 (22.6561, -19.618) -> (21.1656, -19.618)
  spline S196 degree 3 poles (23.308, -19.618) (23.1937, -19.618) (23.1006, -19.5252) (23.1006, -19.4105) knots 0 0 0 0 1 1 1 1
  line L196 (23.1006, -19.4105) -> (23.1006, -18.0086)
  spline S197 degree 3 poles (23.1006, -18.0086) (23.1006, -17.8943) (23.1937, -17.8012) (23.308, -17.8012) knots 0 0 0 0 1 1 1 1
  line L197 (23.308, -17.8012) -> (24.7985, -17.8012)
  spline S198 degree 3 poles (24.7985, -17.8012) (24.9128, -17.8012) (25.0059, -17.8943) (25.0059, -18.0086) knots 0 0 0 0 1 1 1 1
  line L198 (25.0059, -18.0086) -> (25.0059, -19.4105)
  spline S199 degree 3 poles (25.0059, -19.4105) (25.0059, -19.5252) (24.9128, -19.618) (24.7985, -19.618) knots 0 0 0 0 1 1 1 1
  line L199 (24.7985, -19.618) -> (23.308, -19.618)
  spline S200 degree 3 poles (25.4508, -19.618) (25.3361, -19.618) (25.2434, -19.5252) (25.2434, -19.4105) knots 0 0 0 0 1 1 1 1
  line L200 (25.2434, -19.4105) -> (25.2434, -18.0086)
  spline S201 degree 3 poles (25.2434, -18.0086) (25.2434, -17.8943) (25.3361, -17.8012) (25.4508, -17.8012) knots 0 0 0 0 1 1 1 1
  line L201 (25.4508, -17.8012) -> (26.9409, -17.8012)
  spline S202 degree 3 poles (26.9409, -17.8012) (27.0552, -17.8012) (27.1484, -17.8943) (27.1484, -18.0086) knots 0 0 0 0 1 1 1 1
  line L202 (27.1484, -18.0086) -> (27.1484, -19.4105)
  spline S203 degree 3 poles (27.1484, -19.4105) (27.1484, -19.5252) (27.0552, -19.618) (26.9409, -19.618) knots 0 0 0 0 1 1 1 1
  line L203 (26.9409, -19.618) -> (25.4508, -19.618)
  spline S204 degree 3 poles (27.5932, -19.618) (27.4789, -19.618) (27.3858, -19.5252) (27.3858, -19.4105) knots 0 0 0 0 1 1 1 1
  line L204 (27.3858, -19.4105) -> (27.3858, -18.0086)
  spline S205 degree 3 poles (27.3858, -18.0086) (27.3858, -17.8943) (27.4789, -17.8012) (27.5932, -17.8012) knots 0 0 0 0 1 1 1 1
  line L205 (27.5932, -17.8012) -> (29.0834, -17.8012)
  spline S206 degree 3 poles (29.0834, -17.8012) (29.198, -17.8012) (29.2908, -17.8943) (29.2908, -18.0086) knots 0 0 0 0 1 1 1 1
  line L206 (29.2908, -18.0086) -> (29.2908, -19.4105)
  spline S207 degree 3 poles (29.2908, -19.4105) (29.2908, -19.5252) (29.198, -19.618) (29.0834, -19.618) knots 0 0 0 0 1 1 1 1
  line L207 (29.0834, -19.618) -> (27.5932, -19.618)
  spline S208 degree 3 poles (29.7353, -19.618) (29.6213, -19.618) (29.5282, -19.5252) (29.5282, -19.4105) knots 0 0 0 0 1 1 1 1
  line L208 (29.5282, -19.4105) -> (29.5282, -18.0086)
  spline S209 degree 3 poles (29.5282, -18.0086) (29.5282, -17.8943) (29.6213, -17.8012) (29.7353, -17.8012) knots 0 0 0 0 1 1 1 1
  line L209 (29.7353, -17.8012) -> (32.8309, -17.8012)
  spline S210 degree 3 poles (32.8309, -17.8012) (32.9456, -17.8012) (33.0383, -17.8943) (33.0383, -18.0086) knots 0 0 0 0 1 1 1 1
  line L210 (33.0383, -18.0086) -> (33.0383, -19.4105)
  spline S211 degree 3 poles (33.0383, -19.4105) (33.0383, -19.5252) (32.9456, -19.618) (32.8309, -19.618) knots 0 0 0 0 1 1 1 1
  line L211 (32.8309, -19.618) -> (29.7353, -19.618)
  spline S212 degree 3 poles (6.1683, -19.618) (6.0544, -19.618) (5.9612, -19.5252) (5.9612, -19.4105) knots 0 0 0 0 1 1 1 1
  line L212 (5.9612, -19.4105) -> (5.9612, -18.0086)
  spline S213 degree 3 poles (5.9612, -18.0086) (5.9612, -17.8943) (6.0544, -17.8012) (6.1683, -17.8012) knots 0 0 0 0 1 1 1 1
  line L213 (6.1683, -17.8012) -> (7.6588, -17.8012)
  spline S214 degree 3 poles (7.6588, -17.8012) (7.7735, -17.8012) (7.8662, -17.8943) (7.8662, -18.0086) knots 0 0 0 0 1 1 1 1
  line L214 (7.8662, -18.0086) -> (7.8662, -19.4105)
  spline S215 degree 3 poles (7.8662, -19.4105) (7.8662, -19.5252) (7.7735, -19.618) (7.6588, -19.618) knots 0 0 0 0 1 1 1 1
  line L215 (7.6588, -19.618) -> (6.1683, -19.618)
  spline S216 degree 3 poles (2.4208, -19.618) (2.3068, -19.618) (2.2137, -19.5252) (2.2137, -19.4105) knots 0 0 0 0 1 1 1 1
  line L216 (2.2137, -19.4105) -> (2.2137, -18.0086)
  spline S217 degree 3 poles (2.2137, -18.0086) (2.2137, -17.8943) (2.3068, -17.8012) (2.4208, -17.8012) knots 0 0 0 0 1 1 1 1
  line L217 (2.4208, -17.8012) -> (5.5167, -17.8012)
  spline S218 degree 3 poles (5.5167, -17.8012) (5.6307, -17.8012) (5.7238, -17.8943) (5.7238, -18.0086) knots 0 0 0 0 1 1 1 1
  line L218 (5.7238, -18.0086) -> (5.7238, -19.4105)
  spline S219 degree 3 poles (5.7238, -19.4105) (5.7238, -19.5252) (5.6307, -19.618) (5.5167, -19.618) knots 0 0 0 0 1 1 1 1
  line L219 (5.5167, -19.618) -> (2.4208, -19.618)
  spline S220 degree 3 poles (7.2528, -21.7064) (7.1385, -21.7064) (7.0453, -21.6136) (7.0453, -21.499) knots 0 0 0 0 1 1 1 1
  line L220 (7.0453, -21.499) -> (7.0453, -20.097)
  spline S221 degree 3 poles (7.0453, -20.097) (7.0453, -19.9827) (7.1385, -19.8896) (7.2528, -19.8896) knots 0 0 0 0 1 1 1 1
  line L221 (7.2528, -19.8896) -> (8.7432, -19.8896)
  spline S222 degree 3 poles (8.7432, -19.8896) (8.8572, -19.8896) (8.9503, -19.9827) (8.9503, -20.097) knots 0 0 0 0 1 1 1 1
  line L222 (8.9503, -20.097) -> (8.9503, -21.499)
  spline S223 degree 3 poles (8.9503, -21.499) (8.9503, -21.6136) (8.8572, -21.7064) (8.7432, -21.7064) knots 0 0 0 0 1 1 1 1
  line L223 (8.7432, -21.7064) -> (7.2528, -21.7064)
  spline S224 degree 3 poles (9.3952, -21.7064) (9.2809, -21.7064) (9.1877, -21.6136) (9.1877, -21.499) knots 0 0 0 0 1 1 1 1
  line L224 (9.1877, -21.499) -> (9.1877, -20.097)
  spline S225 degree 3 poles (9.1877, -20.097) (9.1877, -19.9827) (9.2809, -19.8896) (9.3952, -19.8896) knots 0 0 0 0 1 1 1 1
  line L225 (9.3952, -19.8896) -> (10.8857, -19.8896)
  spline S226 degree 3 poles (10.8857, -19.8896) (11, -19.8896) (11.0927, -19.9827) (11.0927, -20.097) knots 0 0 0 0 1 1 1 1
  line L226 (11.0927, -20.097) -> (11.0927, -21.499)
  spline S227 degree 3 poles (11.0927, -21.499) (11.0927, -21.6136) (11, -21.7064) (10.8857, -21.7064) knots 0 0 0 0 1 1 1 1
  line L227 (10.8857, -21.7064) -> (9.3952, -21.7064)
  spline S228 degree 3 poles (11.5376, -21.7064) (11.4233, -21.7064) (11.3302, -21.6136) (11.3302, -21.499) knots 0 0 0 0 1 1 1 1
  line L228 (11.3302, -21.499) -> (11.3302, -20.097)
  spline S229 degree 3 poles (11.3302, -20.097) (11.3302, -19.9827) (11.4233, -19.8896) (11.5376, -19.8896) knots 0 0 0 0 1 1 1 1
  line L229 (11.5376, -19.8896) -> (13.0281, -19.8896)
  spline S230 degree 3 poles (13.0281, -19.8896) (13.1424, -19.8896) (13.2352, -19.9827) (13.2352, -20.097) knots 0 0 0 0 1 1 1 1
  line L230 (13.2352, -20.097) -> (13.2352, -21.499)
  spline S231 degree 3 poles (13.2352, -21.499) (13.2352, -21.6136) (13.1424, -21.7064) (13.0281, -21.7064) knots 0 0 0 0 1 1 1 1
  line L231 (13.0281, -21.7064) -> (11.5376, -21.7064)
  spline S232 degree 3 poles (13.68, -21.7064) (13.5657, -21.7064) (13.4726, -21.6136) (13.4726, -21.499) knots 0 0 0 0 1 1 1 1
  line L232 (13.4726, -21.499) -> (13.4726, -20.097)
  spline S233 degree 3 poles (13.4726, -20.097) (13.4726, -19.9827) (13.5657, -19.8896) (13.68, -19.8896) knots 0 0 0 0 1 1 1 1
  line L233 (13.68, -19.8896) -> (15.1705, -19.8896)
  spline S234 degree 3 poles (15.1705, -19.8896) (15.2848, -19.8896) (15.3776, -19.9827) (15.3776, -20.097) knots 0 0 0 0 1 1 1 1
  line L234 (15.3776, -20.097) -> (15.3776, -21.499)
  spline S235 degree 3 poles (15.3776, -21.499) (15.3776, -21.6136) (15.2848, -21.7064) (15.1705, -21.7064) knots 0 0 0 0 1 1 1 1
  line L235 (15.1705, -21.7064) -> (13.68, -21.7064)
  spline S236 degree 3 poles (15.8224, -21.7064) (15.7081, -21.7064) (15.6154, -21.6136) (15.6154, -21.499) knots 0 0 0 0 1 1 1 1
  line L236 (15.6154, -21.499) -> (15.6154, -20.097)
  spline S237 degree 3 poles (15.6154, -20.097) (15.6154, -19.9827) (15.7081, -19.8896) (15.8224, -19.8896) knots 0 0 0 0 1 1 1 1
  line L237 (15.8224, -19.8896) -> (17.3129, -19.8896)
  spline S238 degree 3 poles (17.3129, -19.8896) (17.4272, -19.8896) (17.5204, -19.9827) (17.5204, -20.097) knots 0 0 0 0 1 1 1 1
  line L238 (17.5204, -20.097) -> (17.5204, -21.499)
  spline S239 degree 3 poles (17.5204, -21.499) (17.5204, -21.6136) (17.4272, -21.7064) (17.3129, -21.7064) knots 0 0 0 0 1 1 1 1
  line L239 (17.3129, -21.7064) -> (15.8224, -21.7064)
  spline S240 degree 3 poles (17.9649, -21.7064) (17.8506, -21.7064) (17.7574, -21.6136) (17.7574, -21.499) knots 0 0 0 0 1 1 1 1
  line L240 (17.7574, -21.499) -> (17.7574, -20.097)
  spline S241 degree 3 poles (17.7574, -20.097) (17.7574, -19.9827) (17.8506, -19.8896) (17.9649, -19.8896) knots 0 0 0 0 1 1 1 1
  line L241 (17.9649, -19.8896) -> (19.4553, -19.8896)
  spline S242 degree 3 poles (19.4553, -19.8896) (19.5696, -19.8896) (19.6624, -19.9827) (19.6624, -20.097) knots 0 0 0 0 1 1 1 1
  line L242 (19.6624, -20.097) -> (19.6624, -21.499)
  spline S243 degree 3 poles (19.6624, -21.499) (19.6624, -21.6136) (19.5696, -21.7064) (19.4553, -21.7064) knots 0 0 0 0 1 1 1 1
  line L243 (19.4553, -21.7064) -> (17.9649, -21.7064)
  spline S244 degree 3 poles (20.1073, -21.7064) (19.993, -21.7064) (19.8998, -21.6136) (19.8998, -21.499) knots 0 0 0 0 1 1 1 1
  line L244 (19.8998, -21.499) -> (19.8998, -20.097)
  spline S245 degree 3 poles (19.8998, -20.097) (19.8998, -19.9827) (19.993, -19.8896) (20.1073, -19.8896) knots 0 0 0 0 1 1 1 1
  line L245 (20.1073, -19.8896) -> (21.5978, -19.8896)
  spline S246 degree 3 poles (21.5978, -19.8896) (21.7121, -19.8896) (21.8052, -19.9827) (21.8052, -20.097) knots 0 0 0 0 1 1 1 1
  line L246 (21.8052, -20.097) -> (21.8052, -21.499)
  spline S247 degree 3 poles (21.8052, -21.499) (21.8052, -21.6136) (21.7121, -21.7064) (21.5978, -21.7064) knots 0 0 0 0 1 1 1 1
  line L247 (21.5978, -21.7064) -> (20.1073, -21.7064)
  spline S248 degree 3 poles (22.2497, -21.7064) (22.1354, -21.7064) (22.0423, -21.6136) (22.0423, -21.499) knots 0 0 0 0 1 1 1 1
  line L248 (22.0423, -21.499) -> (22.0423, -20.097)
  spline S249 degree 3 poles (22.0423, -20.097) (22.0423, -19.9827) (22.1354, -19.8896) (22.2497, -19.8896) knots 0 0 0 0 1 1 1 1
  line L249 (22.2497, -19.8896) -> (23.7402, -19.8896)
  spline S250 degree 3 poles (23.7402, -19.8896) (23.8545, -19.8896) (23.9476, -19.9827) (23.9476, -20.097) knots 0 0 0 0 1 1 1 1
  line L250 (23.9476, -20.097) -> (23.9476, -21.499)
  spline S251 degree 3 poles (23.9476, -21.499) (23.9476, -21.6136) (23.8545, -21.7064) (23.7402, -21.7064) knots 0 0 0 0 1 1 1 1
  line L251 (23.7402, -21.7064) -> (22.2497, -21.7064)
  spline S252 degree 3 poles (24.3925, -21.7064) (24.2778, -21.7064) (24.185, -21.6136) (24.185, -21.499) knots 0 0 0 0 1 1 1 1
  line L252 (24.185, -21.499) -> (24.185, -20.097)
  spline S253 degree 3 poles (24.185, -20.097) (24.185, -19.9827) (24.2778, -19.8896) (24.3925, -19.8896) knots 0 0 0 0 1 1 1 1
  line L253 (24.3925, -19.8896) -> (25.8826, -19.8896)
  spline S254 degree 3 poles (25.8826, -19.8896) (25.9969, -19.8896) (26.09, -19.9827) (26.09, -20.097) knots 0 0 0 0 1 1 1 1
  line L254 (26.09, -20.097) -> (26.09, -21.499)
  spline S255 degree 3 poles (26.09, -21.499) (26.09, -21.6136) (25.9969, -21.7064) (25.8826, -21.7064) knots 0 0 0 0 1 1 1 1
  line L255 (25.8826, -21.7064) -> (24.3925, -21.7064)
  spline S256 degree 3 poles (26.5349, -21.7064) (26.4206, -21.7064) (26.3275, -21.6136) (26.3275, -21.499) knots 0 0 0 0 1 1 1 1
  line L256 (26.3275, -21.499) -> (26.3275, -20.097)
  spline S257 degree 3 poles (26.3275, -20.097) (26.3275, -19.9827) (26.4206, -19.8896) (26.5349, -19.8896) knots 0 0 0 0 1 1 1 1
  line L257 (26.5349, -19.8896) -> (28.025, -19.8896)
  spline S258 degree 3 poles (28.025, -19.8896) (28.1397, -19.8896) (28.2325, -19.9827) (28.2325, -20.097) knots 0 0 0 0 1 1 1 1
  line L258 (28.2325, -20.097) -> (28.2325, -21.499)
  spline S259 degree 3 poles (28.2325, -21.499) (28.2325, -21.6136) (28.1397, -21.7064) (28.025, -21.7064) knots 0 0 0 0 1 1 1 1
  line L259 (28.025, -21.7064) -> (26.5349, -21.7064)
  spline S260 degree 3 poles (28.677, -21.7064) (28.563, -21.7064) (28.4699, -21.6136) (28.4699, -21.499) knots 0 0 0 0 1 1 1 1
  line L260 (28.4699, -21.499) -> (28.4699, -20.097)
  spline S261 degree 3 poles (28.4699, -20.097) (28.4699, -19.9827) (28.563, -19.8896) (28.677, -19.8896) knots 0 0 0 0 1 1 1 1
  line L261 (28.677, -19.8896) -> (32.8309, -19.8896)
  spline S262 degree 3 poles (32.8309, -19.8896) (32.9456, -19.8896) (33.0383, -19.9827) (33.0383, -20.097) knots 0 0 0 0 1 1 1 1
  line L262 (33.0383, -20.097) -> (33.0383, -21.499)
  spline S263 degree 3 poles (33.0383, -21.499) (33.0383, -21.6136) (32.9456, -21.7064) (32.8309, -21.7064) knots 0 0 0 0 1 1 1 1
  line L263 (32.8309, -21.7064) -> (28.677, -21.7064)
  spline S264 degree 3 poles (2.4292, -21.7064) (2.3149, -21.7064) (2.2218, -21.6136) (2.2218, -21.499) knots 0 0 0 0 1 1 1 1
  line L264 (2.2218, -21.499) -> (2.2218, -20.097)
  spline S265 degree 3 poles (2.2218, -20.097) (2.2218, -19.9827) (2.3149, -19.8896) (2.4292, -19.8896) knots 0 0 0 0 1 1 1 1
  line L265 (2.4292, -19.8896) -> (6.6005, -19.8896)
  spline S266 degree 3 poles (6.6005, -19.8896) (6.7151, -19.8896) (6.8079, -19.9827) (6.8079, -20.097) knots 0 0 0 0 1 1 1 1
  line L266 (6.8079, -20.097) -> (6.8079, -21.499)
  spline S267 degree 3 poles (6.8079, -21.499) (6.8079, -21.6136) (6.7151, -21.7064) (6.6005, -21.7064) knots 0 0 0 0 1 1 1 1
  line L267 (6.6005, -21.7064) -> (2.4292, -21.7064)
  spline S268 degree 3 poles (6.706, -23.7949) (6.5917, -23.7949) (6.4985, -23.7021) (6.4985, -23.5874) knots 0 0 0 0 1 1 1 1
  line L268 (6.4985, -23.5874) -> (6.4985, -22.1855)
  spline S269 degree 3 poles (6.4985, -22.1855) (6.4985, -22.0708) (6.5917, -21.9781) (6.706, -21.9781) knots 0 0 0 0 1 1 1 1
  line L269 (6.706, -21.9781) -> (8.1964, -21.9781)
  spline S270 degree 3 poles (8.1964, -21.9781) (8.3107, -21.9781) (8.4035, -22.0708) (8.4035, -22.1855) knots 0 0 0 0 1 1 1 1
  line L270 (8.4035, -22.1855) -> (8.4035, -23.5874)
  spline S271 degree 3 poles (8.4035, -23.5874) (8.4035, -23.7021) (8.3107, -23.7949) (8.1964, -23.7949) knots 0 0 0 0 1 1 1 1
  line L271 (8.1964, -23.7949) -> (6.706, -23.7949)
  spline S272 degree 3 poles (8.8484, -23.7949) (8.7341, -23.7949) (8.6409, -23.7021) (8.6409, -23.5874) knots 0 0 0 0 1 1 1 1